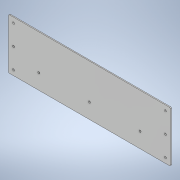
# Autodesk Inventor part: Platform side 1
Saved by Autodesk Inventor 2020 (Build 240168000, 168)
## iProperties
Created: 2022-07-05
Part Number: Platform side 1
Material: Generic
Document SubType Name: Sheet Metal
Designer: karimi2
Density: 1 g/cm^3
Sheet Metal Rule: Default_mm
Appearance: Aluminum - Dark
Author: karimi2
Autodesk Inventor part; units mm, degrees
ref_plane "YZ Plane" through (0, 0, 0) normal (1, 0, 0) x (0, 1, 0)
ref_plane "XZ Plane" through (0, 0, 0) normal (0, 1, 0) x (-1, 0, 0)
ref_plane "XY Plane" through (0, 0, 0) normal (0, 0, 1) x (1, 0, 0)
sketch "Sketch1" plane through (0, 0, 0) normal (0, 0, 1) x (1, 0, 0)
  line L0 (160, -50) -> (-160, -50)
  line L1 (-160, -50) -> (-160, 50)
  line L2 (-160, 50) -> (160, 50)
  line L3 (160, 50) -> (160, -50)
  circle A0 centre (-100, -20) radius 2
  circle A1 centre (0, -20) radius 2
  circle A2 centre (100, -20) radius 2
  circle A3 centre (-150, 40) radius 2
  circle A4 centre (-150, 0) radius 2
  circle A5 centre (-150, -40) radius 2
  circle A6 centre (150, 40) radius 2
  circle A7 centre (150, 0) radius 2
  circle A8 centre (150, -40) radius 2
  point P0 (0, 0)
  dimension "d0" = 320
  dimension "d1" = 100
  dimension "d8" = 60
  dimension "d9" = 30
  dimension "d10" = 4
  dimension "d11" = 60
  dimension "d12" = 30
  dimension "d13" = 10
  dimension "d14" = 10
  dimension "d15" = 10
  dimension "d16" = 10
  dimension "d17" = 10
  dimension "d18" = 4
  dimension "d21" = 160
  dimension "d22" = 50
  dimension "d23" = 160
  measures "d0" distance of L1.end L2.end
  measures "d1" distance of L2.end L0.start
  measures "d8" distance from line of L1 A0.centre
  measures "d9" distance from line of L0 A0.centre
  measures "d10" diameter of A0
  measures "d11" distance from line of L3 A2.centre
  measures "d12" distance from line of L0 A2.centre
  measures "d13" distance from line of L1 A3.centre
  measures "d14" distance from line of L2 A3.centre
  measures "d15" distance from line of L0 A5.centre
  measures "d16" distance from line of L1 A5.centre
  measures "d17" distance from line of L3 A6.centre
  measures "d18" diameter of A3
  measures "d21" distance from line of point (0, 0) L3
  measures "d22" distance from line of point (0, 0) L2
  measures "d23" distance from line of A1.centre L3
extrude "Plate1" add sketch "Sketch1" along normal blind 2
fillet "Fillet1" radius 2 4 edges at (160, 50, 1) (160, -50, 1) (-160, 50, 1) (-160, -50, 1)
equation "\"d19\" = Thickness"
equation "\"BendRadius\" = Thickness"
equation "\"BendReliefWidth\" = Thickness"
equation "\"BendReliefDepth\" = 0.5 * Thickness"
equation "\"CornerReliefSize\" = 4 * Thickness"
equation "\"MinimumRemnant\" = 2 * Thickness"
equation "\"TransitionRadius\" = BendRadius"
equation "\"JacobiRadiusSize\" = BendRadius"
equation "\"GapSize\" = Thickness"
equation "\"Thickness\" = 2"
body "Solid1"
